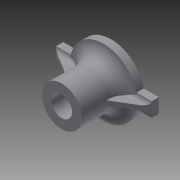
# Autodesk Inventor part: propeller-holder
Saved by Autodesk Inventor 2014 SP2 (Build 180247200, 247)
## iProperties
Created: 2016-10-04
Part Number: propeller-holder
Material: 一般
Document SubType Name: Modeling
Designer: hide
Density: 1 g/cm^3
Appearance: 既定
Author: hide
Autodesk Inventor part; units mm, degrees
ref_plane "YZ Plane" through (0, 0, 0) normal (1, 0, 0) x (0, 1, 0)
ref_plane "XZ Plane" through (0, 0, 0) normal (0, 1, 0) x (-1, 0, 0)
ref_plane "XY Plane" through (0, 0, 0) normal (0, 0, 1) x (1, 0, 0)
sketch "スケッチ2" plane through (0, 0, 0) normal (0, 1, 0) x (-1, 0, 0)
  circle A0 centre (0, 0) radius 2.15
  circle A1 centre (0, 0) radius 4.15
  dimension "d5" = 2
  dimension "d6" = 4.3
  constraints: 2 centre point, 2 coincident
  measures "d5" radial gap between concentric circles of A0 A1
  measures "d6" diameter of A0
extrude "押し出し1" add sketch "スケッチ2" along normal blind 10.3
sketch "スケッチ3" plane through (0, 0, 0) normal (1, 0, 0) x (0, 1, 0)
  circle A0 centre (3.8, 0) radius 0.75
  point P0 (0, 0)
  dimension "d9" = 1.5
  dimension "d10" = 0
  dimension "d11" = 3.8
  constraints: 1 centre point
  measures "d9" diameter of A0
  measures "d10" vertical distance of point (0, 0) A0.centre
  measures "d11" distance of point (0, 0) A0.centre
extrude "押し出し2" cut sketch "スケッチ3" against normal blind 9.3
sketch "スケッチ4" plane through (0, 10.3, 0) normal (0, 1, 0) x (1, 0, 0)
  circle A0 centre (0, 0) radius 2.15 projected
  circle A1 centre (0, 0) radius 4.15 projected
  line L0 (-7, 7) -> (7, 7)
  line L1 (7, 7) -> (7, -7)
  line L2 (7, -7) -> (-7, -7)
  line L3 (-7, -7) -> (-7, 7)
  dimension "d19" = 14
  dimension "d20" = 7
  dimension "d22" = 14
  dimension "d23" = 7
  constraints: 8 end point, 2 parallel, 1 horizontal, 1 perpendicular
  measures "d19" distance of L2.end L0.start
  measures "d20" distance from line of A0.centre L0
  measures "d22" distance between parallel lines of L3 L1
  measures "d23" distance from line of A0.centre L3
extrude "押し出し3" add sketch "スケッチ4" against normal blind 1.6 contours L0 L1 L2 L3
fillet "フィレット4" radius 7 4 edges at (7, 9.5, 7) (7, 9.5, -7) (-7, 9.5, 7) (-7, 9.5, -7)
sketch "スケッチ9" plane through (0, 10.3, 0) normal (0, 1, 0) x (1, 0, 0)
  circle A0 centre (0, 0) radius 7 projected
  line L0 (-4, 1.5) -> (-10, 1.5)
  line L1 (-10, 1.5) -> (-10, -1.5)
  line L2 (-10, -1.5) -> (-4, -1.5)
  line L3 (-4, -1.5) -> (-4, 1.5)
  dimension "d56" = 4
  dimension "d57" = 6
  dimension "d63" = 3
  dimension "d64" = 1.5
  constraints: 8 end point, 2 parallel, 1 horizontal, 1 perpendicular
  measures "d56" distance from line of A0.centre L3
  measures "d57" distance of L0.start L0.end
  measures "d63" distance of L0.end L1.end
  measures "d64" distance from line of A0.centre L0
extrude "押し出し8" add sketch "スケッチ9" against normal blind 1.5 contours L0 L3 L2 A0 | A0 L2 L1 L0 picked at (-4.994, -0.1678)
mirror "ミラー1" about plane through (0, 0, 0) normal (1, 0, 0) of "押し出し8"
sketch "スケッチ13" plane through (0, 0, 0) normal (0, 0, 1) x (1, 0, 0)
  line L0 (-6.8374, 10.3) -> (-6.8374, 8.8) projected
  line L1 (-10, 10.3) -> (-6.8374, 10.3) projected
  line L2 (-10, 10.3) -> (-10, 8.8) projected
  line L3 (-6.8374, 8.8) -> (-10, 8.8) projected
  line L4 (-10, 8.8) -> (-4.0073, 5.1965)
  line L5 (-4.0073, 5.1965) -> (-4.0073, 8.8)
  line L6 (-4.0073, 8.8) -> (-10, 8.8)
  point P0 (0, 0)
  constraints: 6 end point, 2 perpendicular
extrude "押し出し12" add sketch "スケッチ13" along normal mid plane 1 contours L6 L5 L4 L3
sketch "スケッチ14" plane through (0, 10.3, 0) normal (0, 1, 0) x (1, 0, 0)
  circle A0 centre (0, 0) radius 2.15 projected
  arc A1 (-6.8374, -1.5) -> (6.8374, -1.5) centre (0, 0) ccw projected
  line L0 (3.926, 0) -> (1.963, -3.4)
  line L1 (1.963, -3.4) -> (-1.963, -3.4)
  line L2 (-1.963, -3.4) -> (-3.926, 0)
  line L3 (-3.926, 0) -> (-1.963, 3.4)
  line L4 (-1.963, 3.4) -> (1.963, 3.4)
  line L5 (1.963, 3.4) -> (3.926, 0)
  dimension "d76" = 6.8
  constraints: 12 end point, 1 coincident, 13 other
  measures "d76" distance between parallel lines of L1 L4
extrude "押し出し13" add sketch "スケッチ14" along normal blind 1.5
mirror "ミラー2" about plane through (0, 0, 0) normal (1, 0, 0) of "押し出し12"
fillet "フィレット5" radius 1 4 edges at (-8.4911, 8.8, -0.5) (-8.4911, 8.8, 0.5) (8.4911, 8.8, 0.5) (8.4911, 8.8, -0.5)
fillet "フィレット6" radius 2.8 2 edges at (0, 8.7, 4.15) (0, 8.7, -4.15)
equation "\"d20\" = 0.5 * d19"
equation "\"d22\" = d19"
equation "\"d23\" = 0.5 * d22"
equation "\"d64\" = 0.5 * d63"
